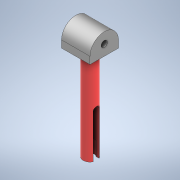
# Autodesk Inventor part: pist
Saved by Autodesk Inventor 2022 (Build 260153000, 153)
## iProperties
Created: 2022-11-09
Part Number: pist
Material: Generic
Document SubType Name: Modeling
Designer: matys
Density: 1 g/cm^3
Appearance: Default
Author: matys
Autodesk Inventor part; units mm, degrees
ref_plane "YZ Plane" through (0, 0, 0) normal (1, 0, 0) x (0, 1, 0)
ref_plane "XZ Plane" through (0, 0, 0) normal (0, 1, 0) x (-1, 0, 0)
ref_plane "XY Plane" through (0, 0, 0) normal (0, 0, 1) x (1, 0, 0)
sketch "Sketch1" plane through (0, 0, 0) normal (0, 1, 0) x (-1, 0, 0)
  circle A0 centre (0, 0) radius 2.4
  dimension "d0" = 4.8
  constraints: 1 centre point, 1 coincident
  measures "d0" diameter of A0
extrude "Extrusion1" add sketch "Sketch1" along normal blind 33
sketch "Sketch2" plane through (0, 33, 0) normal (0, 1, 0) x (1, 0, 0)
  line L0 (-5, 0) -> (5, 0)
  line L1 (-5, 0) -> (-5, -5)
  line L2 (-5, -5) -> (5, -5)
  line L3 (5, -5) -> (5, 0)
  line L4 (-5, 0) -> (-5, 5)
  line L5 (-5, 5) -> (5, 5)
  line L6 (5, 5) -> (5, 0)
  point P0 (0, 0)
  dimension "d4" = 10
  dimension "d5" = 5
  dimension "d6" = 5
  constraints: 14 end point, 4 perpendicular, 2 point on line, 1 vertical
  measures "d4" distance of L0.start L0.end
  measures "d5" distance of L0.start L1.end
  measures "d6" distance of L0.start L4.end
extrude "Extrusion2" add sketch "Sketch2" along normal blind 7.5
fillet "Fillet1" radius 5 2 edges at (0, 40.5, 5) (0, 40.5, -5)
sketch "Sketch3" plane through (5, 33, 5) normal (1, 0, 0) x (0, 0, -1)
  line L0 (10, 0) -> (0, 0) projected
  line L1 (5, 0) -> (5, 7.5)
  arc A0 (10, 2.5) -> (0, 2.5) centre (5, 2.5) ccw projected
  line L2 (5, 0) -> (5, 3.75)
  circle A1 centre (5, 3.75) radius 1.1
  point P0 (5, -33)
  dimension "d10" = 2.2
  constraints: 4 end point, 2 midpoint, 1 centre point, 1 coincident, 1 point on circle, 1 vertical
  measures "d10" diameter of A1
extrude "Extrusion3" cut sketch "Sketch3" against normal through all
sketch "Sketch5" plane through (0, 0, 0) normal (0, -1, 0) x (1, 0, 0)
  circle A0 centre (0, 0) radius 2.4
  circle A1 centre (0, 0) radius 1.5
  dimension "d19" = 3
  constraints: 2 centre point, 2 coincident
  measures "d19" diameter of A1
extrude "Extrusion5" cut sketch "Sketch5" against normal blind 5 contours A1
sketch "Sketch6" plane through (5, 33, 5) normal (1, 0, 0) x (0, 0, -1)
  line L0 (5, -33) -> (5, -32)
  line L1 (5, -32) -> (5, -24)
  line L2 (5, -24) -> (5, -32) construction
  line L3 (3.95, -25.05) -> (3.95, -30.95)
  line L4 (6.05, -30.95) -> (6.05, -25.05)
  arc A0 (6.05, -25.05) -> (3.95, -25.05) centre (5, -25.05) ccw
  arc A1 (3.95, -30.95) -> (6.05, -30.95) centre (5, -30.95) ccw
  line L5 (5, -33) -> (5, -24) construction
  line L6 (7.4, -33) -> (2.6, -33) projected
  line L7 (3.95, -31.95) -> (3.95, -25.05)
  line L8 (6.05, -25.05) -> (6.05, -31.95)
  arc A2 (3.95, -31.95) -> (6.05, -31.95) centre (5, -31.95) ccw
  arc A3 (6.05, -25.05) -> (3.95, -25.05) centre (5, -25.05) ccw
  line L9 (3.95, -31.95) -> (3.95, -33)
  line L10 (6.05, -31.95) -> (6.05, -33)
  line L11 (3.95, -33) -> (6.05, -33)
  line L12 (5, -24) -> (5, 0)
  line L13 (7.4, 0) -> (2.6, 0) projected
  line L14 (5, 0) -> (5, -33)
  line L15 (5, -16.5) -> (7.4, -16.5)
  line L16 (7.4, -33) -> (7.4, 0) projected
  line L17 (5, -16.5) -> (5, -28) construction
  line L18 (3.95, -17.55) -> (3.95, -26.95)
  line L19 (6.05, -26.95) -> (6.05, -17.55)
  arc A4 (6.05, -17.55) -> (3.95, -17.55) centre (5, -17.55) ccw
  arc A5 (3.95, -26.95) -> (6.05, -26.95) centre (5, -26.95) ccw
  point P0 (5, -28.5)
  point P1 (6.05, -30.95)
  point P2 (5, -22.25)
  dimension "d22" = 1
  dimension "d23" = 8
  dimension "d24" = 2.1
  constraints: 40 end point, 18 point on circle, 13 tangent, 9 point on line, 6 centre point, 6 midpoint, 4 collinear, 3 parallel, 2 perpendicular, 2 vertical
  measures "d22" distance of L0.start L0.end
  measures "d23" distance of L0.end L1.end
  measures "d24" diameter of A1
extrude "Extrusion6" cut sketch "Sketch6" against normal through all contours A2 L7 A1 L0 | A2 L10 L6 | L6 L9 A2 | L0 A1 L8 A2 | A1 L3 A5 L1 | L1 A5 L4 A1 | A5 L3 A0 L1 | L1 A0 L4 A5 | L12 A4 L19 A0 | A0 L18 A4 L12
body "Solid1"
